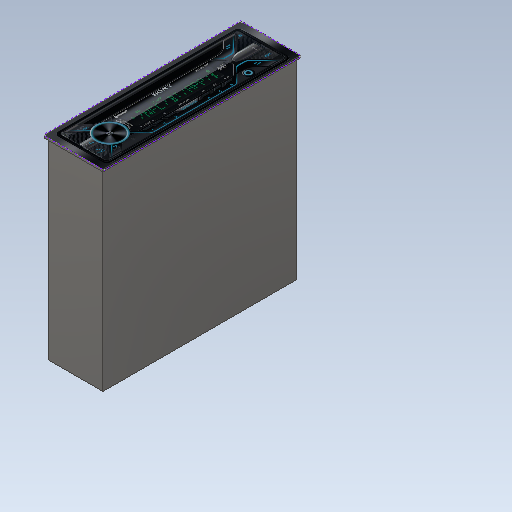
# Autodesk Inventor part: stereo
Saved by Autodesk Inventor 2021 (Build 250183000, 183)
## iProperties
Created: 2020-05-18
Part Number: stereo
Material: Stainless Steel
Document SubType Name: Modeling
Designer: Johansson
Density: 8 g/cm^3
Appearance: Semi-Polished
Author: Johansson
Autodesk Inventor part; units mm, degrees
ref_plane "YZ Plane" through (0, 0, 0) normal (1, 0, 0) x (0, 1, 0)
ref_plane "XZ Plane" through (0, 0, 0) normal (0, 1, 0) x (-1, 0, 0)
ref_plane "XY Plane" through (0, 0, 0) normal (0, 0, 1) x (1, 0, 0)
sketch "Sketch1" plane through (0, 0, 0) normal (0, 1, 0) x (-1, 0, 0)
  line L0 (-25, 89) -> (25, 89)
  line L1 (25, 89) -> (25, -89)
  line L2 (25, -89) -> (-25, -89)
  line L3 (-25, -89) -> (-25, 89)
  line L4 (-25, 89) -> (25, -89) construction
  line L5 (25, 89) -> (-25, -89) construction
  point P0 (0, 0)
  dimension "d0" = 178
  dimension "d1" = 50
  constraints: 12 end point, 2 midpoint, 2 parallel, 1 horizontal, 1 perpendicular
  measures "d0" distance of L0.end L1.end
  measures "d1" distance of L1.end L2.end
extrude "Extrusion1" add sketch "Sketch1" along normal blind 177
sketch "Sketch2" plane through (0, 177, 0) normal (0, 1, 0) x (1, 0, 0)
  line L0 (27, -91) -> (-27, -91)
  line L1 (-27, -91) -> (-27, 91)
  line L2 (-27, 91) -> (27, 91)
  line L3 (27, 91) -> (27, -91)
  line L4 (27, -91) -> (-27, 91) construction
  line L5 (-27, -91) -> (27, 91) construction
  line L6 (25, 89) -> (-25, 89) projected
  line L7 (-25, 89) -> (-25, -89) projected
  point P0 (0, 0)
  dimension "d4" = 2
  dimension "d5" = 2
  constraints: 12 end point, 2 midpoint, 2 parallel, 1 horizontal, 1 perpendicular
  measures "d4" distance between parallel lines of L6 L2
  measures "d5" distance between parallel lines of L7 L1
extrude "Extrusion2" add sketch "Sketch2" along normal blind 2
sketch "Sketch3" plane through (0, 179, 0) normal (0, 1, 0) x (1, 0, 0)
  line L0 (-28.0615, -91.1516) -> (-28.0615, 90.8484) construction
  line L1 (-28.0615, 90.8484) -> (28.3189, 90.8484) construction
  line L2 (28.3189, 90.8484) -> (28.3189, -91.1516) construction
  line L3 (28.3189, -91.1516) -> (-28.0615, -91.1516) construction
  constraints: 2 other
equation "\"d0\" = l_stereo"
equation "\"d1\" = w_stereo"
equation "\"d2\" = d_stereo"
equation "\"d5\" = d4"
equation "\"wl_panel\" = 285"
equation "\"t_panel\" = 8"
equation "\"r_button\" = 8"
equation "\"l_stereo\" = 178"
equation "\"w_stereo\" = 50"
equation "\"d_stereo\" = 177"
equation "\"w_label\" = 15"
equation "\"r_labelscrew\" = 2.5"
equation "\"ro_labelscrew\" = 5"
equation "\"l_buttontobutton\" = 25"
equation "\"r_usboutlet\" = 29"
equation "\"l_fastener_button\" = 19"
body "Solid1"
